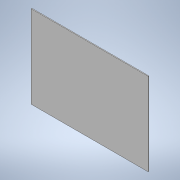
# Autodesk Inventor part: A4
Saved by Autodesk Inventor 2021 (Build 250183000, 183)
## iProperties
Created: 2024-06-01
Part Number: A4
Material: Generic
Document SubType Name: Modeling
Designer: user
Density: 1 g/cm^3
Appearance: Default
Author: user
Autodesk Inventor part; units mm, degrees
ref_plane "YZ Plane" through (0, 0, 0) normal (1, 0, 0) x (0, 1, 0)
ref_plane "XZ Plane" through (0, 0, 0) normal (0, 1, 0) x (-1, 0, 0)
ref_plane "XY Plane" through (0, 0, 0) normal (0, 0, 1) x (1, 0, 0)
sketch "Sketch1" plane through (0, 0, 0) normal (0, 0, 1) x (1, 0, 0)
  line L0 (-177.0096, 123.4211) -> (119.9904, 123.4211)
  line L1 (119.9904, 123.4211) -> (119.9904, -86.5789)
  line L2 (119.9904, -86.5789) -> (-177.0096, -86.5789)
  line L3 (-177.0096, -86.5789) -> (-177.0096, 123.4211)
  point P0 (0, 0)
  dimension "d0" = 210
  dimension "d1" = 297
  constraints: 8 end point, 2 parallel, 1 horizontal, 1 perpendicular
  measures "d0" distance of L2.end L0.start
  measures "d1" distance of L0.start L0.end
extrude "Extrusion1" add sketch "Sketch1" along normal blind 2
body "Solid1"
